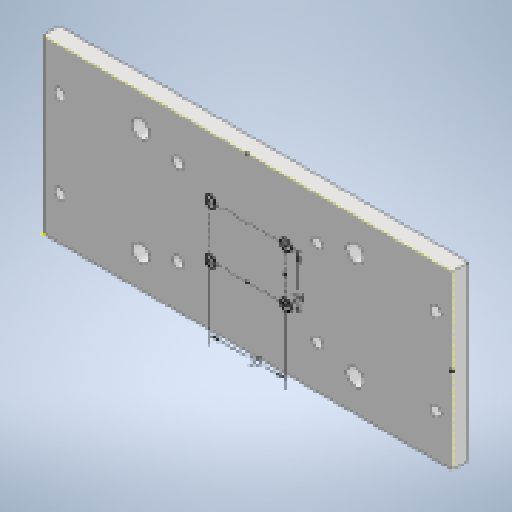
# Autodesk Inventor part: Spindle_Mounting_Plate
Saved by Autodesk Inventor 2023 (Build 270158000, 158)
## iProperties
Created: 2022-05-06
Part Number: Spindle_Mounting_Plate
Material: Generic
Document SubType Name: Modeling
Designer: plebbb
Density: 1 g/cm^3
Appearance: Default
Mass: 105.658 g
Surface Area: 333.842 cm^2
Volume: 105.658 cm^3
Author: plebbb
Autodesk Inventor part; units mm, degrees
ref_plane "YZ Plane" through (0, 0, 0) normal (1, 0, 0) x (0, 1, 0)
ref_plane "XZ Plane" through (0, 0, 0) normal (0, 1, 0) x (-1, 0, 0)
ref_plane "XY Plane" through (0, 0, 0) normal (0, 0, 1) x (1, 0, 0)
sketch "Sketch1" plane through (0, 0, 0) normal (0, 0, 1) x (1, 0, 0)
  line L0 (0, 0) -> (190.5, 0)
  line L1 (190.5, 0) -> (190.5, 80)
  line L2 (190.5, 80) -> (0, 80)
  line L3 (0, 80) -> (0, 0)
  dimension "d0" = 80
  dimension "d1" = 190.5
  constraints: 8 end point, 2 parallel, 1 horizontal, 1 perpendicular
  measures "d0" distance of L0.end L1.end
  measures "d1" distance of L1.end L2.end
extrude "Extrusion1" add sketch "Sketch1" along normal blind 7.62
sketch "Sketch2" plane through (0, 0, 7.62) normal (0, 0, 1) x (1, 0, 0)
  line L0 (45.25, 15) -> (145.25, 15) construction
  line L1 (145.25, 15) -> (145.25, 65) construction
  line L2 (145.25, 65) -> (45.25, 65) construction
  line L3 (45.25, 65) -> (45.25, 15) construction
  line L4 (190.5, 80) -> (0, 80) construction
  line L5 (190.5, 0) -> (190.5, 80) construction
  circle A0 centre (45.25, 65) radius 4
  circle A1 centre (145.25, 65) radius 4
  circle A2 centre (45.25, 15) radius 4
  circle A3 centre (145.25, 15) radius 4
  point P0 (0, 0)
  point P1 (95.25, 65)
  point P2 (95.25, 80)
  point P3 (145.25, 40)
  point P4 (190.5, 40)
  dimension "d4" = 100
  dimension "d5" = 50
  dimension "d6" = 8
  constraints: 8 end point, 4 centre point, 4 coincident, 4 midpoint, 3 equal radius, 2 parallel, 1 horizontal, 1 horizontal alignment, 1 perpendicular, 1 vertical alignment
  measures "d4" distance of L1.end L2.end
  measures "d5" distance of L0.end L1.end
  measures "d6" diameter of A0
extrude "Extrusion2" cut sketch "Sketch2" against normal up to surface (7.62 mm away)
sketch "Sketch3" plane through (0, 0, 7.62) normal (0, 0, 1) x (1, 0, 0)
  line L0 (7.75, 20) -> (62.75, 20) construction
  line L1 (62.75, 20) -> (62.75, 60) construction
  line L2 (62.75, 60) -> (7.75, 60) construction
  line L3 (7.75, 60) -> (7.75, 20) construction
  circle A0 centre (7.75, 60) radius 2.5
  circle A1 centre (62.75, 60) radius 2.5
  circle A2 centre (7.75, 20) radius 2.5
  circle A3 centre (62.75, 20) radius 2.5
  line L4 (190.5, 80) -> (0, 80) construction
  line L5 (95.25, 80) -> (95.25, 0)
  line L6 (0, 0) -> (190.5, 0) construction
  circle A4 centre (182.75, 60) radius 2.5
  circle A5 centre (127.75, 60) radius 2.5
  circle A6 centre (182.75, 20) radius 2.5
  circle A7 centre (127.75, 20) radius 2.5
  point P0 (62.75, 40)
  point P1 (35.25, 60)
  point P2 (95.25, 40)
  dimension "d9" = 5
  dimension "d10" = 55
  dimension "d11" = 40
  dimension "d12" = 60
  constraints: 10 end point, 8 centre point, 5 midpoint, 4 coincident, 4 symmetric about line, 3 equal radius, 2 parallel, 2 perpendicular, 1 horizontal, 1 horizontal alignment, 4 other
  measures "d9" diameter of A0
  measures "d10" distance of L1.end L2.end
  measures "d11" distance of L0.end L1.end
  measures "d12" distance from line of L5 point (35.25, 60)
extrude "Extrusion3" cut sketch "Sketch3" against normal up to surface (7.62 mm away)
sketch "Sketch4" plane through (0, 0, 7.62) normal (0, 0, 1) x (1, 0, 0)
  line L0 (77.75, 42) -> (112.75, 42) construction
  line L1 (112.75, 42) -> (112.75, 66) construction
  line L2 (112.75, 66) -> (77.75, 66) construction
  line L3 (77.75, 66) -> (77.75, 42) construction
  circle A0 centre (112.75, 42) radius 2.5
  circle A1 centre (112.75, 66) radius 2.5
  circle A2 centre (77.75, 66) radius 2.5
  circle A3 centre (77.75, 42) radius 2.5
  line L4 (190.5, 80) -> (0, 80) construction
  line L5 (190.5, 0) -> (190.5, 80) construction
  point P0 (0, 0)
  point P1 (95.25, 42)
  point P2 (95.25, 80)
  point P3 (190.5, 40)
  point P4 (112.75, 54)
  dimension "d15" = 5
  dimension "d16" = 35
  dimension "d17" = 24
  dimension "d18" = 14
  constraints: 8 end point, 4 centre point, 4 coincident, 4 midpoint, 3 equal radius, 2 parallel, 1 horizontal, 1 perpendicular, 1 vertical alignment
  measures "d15" diameter of A0
  measures "d16" distance of L0.start L0.end
  measures "d17" distance of L0.end L1.end
  measures "d18" distance between parallel lines of L4 L2
extrude "Extrusion4" cut sketch "Sketch4" against normal up to surface (7.62 mm away)
body "Solid1"
